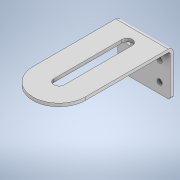
# Autodesk Inventor part: Pieza6
Saved by Autodesk Inventor 2021 (Build 250183000, 183)
## iProperties
Created: 2022-09-12
Part Number: Pieza6
Material: Genérico
Document SubType Name: Modeling
Designer: arthu
Density: 1 g/cm^3
Appearance: Valor por defecto
Author: arthu
Autodesk Inventor part; units mm, degrees
ref_plane "YZ Plane" through (0, 0, 0) normal (1, 0, 0) x (0, 1, 0)
ref_plane "XZ Plane" through (0, 0, 0) normal (0, 1, 0) x (-1, 0, 0)
ref_plane "XY Plane" through (0, 0, 0) normal (0, 0, 1) x (1, 0, 0)
sketch "Boceto1" plane through (0, 0, 0) normal (0, 0, 1) x (1, 0, 0)
  line L0 (0, 0) -> (-50, 0)
  line L1 (-50, 0) -> (-50, 125)
  line L2 (0, 125) -> (0, 0)
  arc A0 (0, 125) -> (-50, 125) centre (-25, 125) ccw
  arc A1 (-20, 125) -> (-30, 125) centre (-25, 125) ccw
  line L3 (-25, 67.5) -> (-25, 60)
  arc A2 (-30, 60) -> (-20, 60) centre (-25, 60) ccw
  line L4 (-30, 60) -> (-30, 125)
  line L5 (-20, 60) -> (-20, 125)
  line L6 (0, 0) -> (-50, 0)
  line L7 (-50, 0) -> (-50, 38.1)
  line L8 (-50, 38.1) -> (0, 38.1)
  line L9 (0, 38.1) -> (0, 0)
  line L10 (-10, 28.1) -> (-40, 28.1)
  line L11 (-40, 28.1) -> (-40, 10)
  line L12 (-40, 10) -> (-10, 10)
  line L13 (-10, 10) -> (-10, 28.1)
  circle A3 centre (-40, 28.1) radius 2.5
  circle A4 centre (-10, 28.1) radius 2.5
  circle A5 centre (-40, 10) radius 2.5
  circle A6 centre (-10, 10) radius 2.5
  point P0 (-12.5, 10)
  point P1 (-10, 12.5)
  point P2 (-10, 25.6)
  point P3 (-12.5, 28.1)
  point P4 (-37.5, 28.1)
  point P5 (-40, 25.6)
  point P6 (-40, 12.5)
  point P7 (-37.5, 10)
  dimension "d2" = 10
  dimension "d3" = 65
  dimension "d4" = 10
  dimension "d5" = 38.1
  dimension "d6" = 10
  dimension "d7" = 5
  dimension "d8" = 5
  dimension "d9" = 5
  dimension "d10" = 5
  constraints: 28 end point, 7 centre point, 6 coincident, 6 point on circle, 6 tangent, 5 parallel, 3 perpendicular, 2 horizontal, 1 point on line, 1 vertical, 3 other
  measures "d2" diameter of A1
  measures "d3" distance of A1.centre L3.end
  measures "d4" diameter of A2
  measures "d5" distance of L6.end L7.end
  measures "d6" distance between parallel lines of L8 L10
  measures "d7" diameter of A3
  measures "d8" diameter of A4
  measures "d9" diameter of A5
  measures "d10" diameter of A6
extrude "Extrusión1" add sketch "Boceto1" along normal blind 3 contours L0 L1 L8 L2 | L8 L1 A0 L2 | L5 A2 L4 A1 | A3 L11 L10 | L10 L11 A3 | L10 A4 L13 A6 L12 A5 L11 A3 | A4 L13 L10 | L10 L13 A4 | A5 L12 L11 | L11 L12 A5 | A6 L12 L13 | L13 L12 A6
fillet "Empalme1" radius 2 2 edges at (0, 0, 1.5) (-50, 0, 1.5)
extrude "Extrusión2" cut sketch "Boceto1" along normal blind 3 contours L5 A2 L4 A1 | A3 L11 L10 | L10 L11 A3 | A4 L13 L10 | L10 L13 A4 | A5 L12 L11 | L11 L12 A5 | A6 L12 L13 | L13 L12 A6
bend part "Pieza de plegado1" radius 5 angle 90 line through (-50, 38.1, 0) along (1, 0, 0) centre toward (0, 0, 1) moving side (0, 1, 0) both sides no
